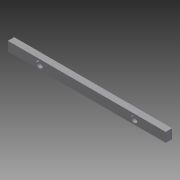
# Autodesk Inventor part: FRC Axle Base
Saved by Autodesk Inventor 2012 (Build 160160000, 160)
## iProperties
Created: 2012-01-10
Part Number: FRC Axle Base
Material: Default
Document SubType Name: Modeling
Designer: Logan
Density: 1 g/cm^3
Author: Logan
Autodesk Inventor part; units mm, degrees
ref_plane "YZ Plane" through (0, 0, 0) normal (1, 0, 0) x (0, 1, 0)
ref_plane "XZ Plane" through (0, 0, 0) normal (0, 1, 0) x (-1, 0, 0)
ref_plane "XY Plane" through (0, 0, 0) normal (0, 0, 1) x (1, 0, 0)
sketch "Sketch1" plane through (0, 0, 0) normal (0, 0, 1) x (1, 0, 0)
  line L0 (634.9648, 0) -> (-0.0352, 0)
  line L1 (-0.0352, 0) -> (-0.0352, 38.1)
  line L2 (-0.0352, 38.1) -> (634.9648, 38.1)
  line L3 (634.9648, 38.1) -> (634.9648, 0)
  circle A0 centre (126.9648, 19.05) radius 12.7
  circle A1 centre (507.9648, 19.05) radius 12.7
  point P0 (-0.0352, 19.05)
  dimension "d2" = 635
  dimension "d3" = 38.1
  dimension "d4" = 25.4
  dimension "d5" = 25.4
  dimension "d6" = 381
  dimension "d7" = 127
  constraints: 8 end point, 2 centre point, 2 horizontal alignment, 2 parallel, 1 horizontal, 1 midpoint, 1 perpendicular
  measures "d2" distance of L0.start L0.end
  measures "d3" distance between parallel lines of L0 L2
  measures "d4" diameter of A0
  measures "d5" diameter of A1
  measures "d6" distance of A1.centre A0.centre
  measures "d7" distance of point (-0.035, 19.05) A0.centre
extrude "Extrusion1" add sketch "Sketch1" along normal blind 25.4 contours L0 L1 L2 L3 | A0 | A1
sketch "Sketch2" plane through (0, 0, 25.4) normal (0, 0, 1) x (1, 0, 0)
  line L0 (-0.0352, 0) -> (-0.0352, 38.1) projected
  circle A0 centre (126.9648, 19.05) radius 12.7
  circle A1 centre (507.9648, 19.05) radius 12.7
  point P0 (0, 0)
  point P1 (-0.0352, 19.05)
  dimension "d10" = 381
  dimension "d11" = 127
  dimension "d12" = 25.4
  dimension "d13" = 25.4
  constraints: 2 centre point, 2 horizontal alignment, 1 midpoint
  measures "d10" distance of A1.centre A0.centre
  measures "d11" distance from line of L0 A0.centre
  measures "d12" diameter of A0
  measures "d13" diameter of A1
extrude "Extrusion2" cut sketch "Sketch2" against normal blind 12.7
equation "\"d5\" = d4"
equation "\"d13\" = d12"
body "Solid1"
